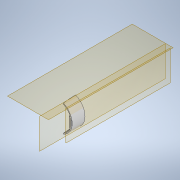
# Autodesk Inventor part: Deckel_Parachute_5_2
Saved by Autodesk Inventor 2020 (Build 240168000, 168)
## iProperties
Created: 2022-01-25
Part Number: Deckel_Parachute_5_2
Material: Generisch
Document SubType Name: Modeling
Designer: sp
Density: 1 g/cm^3
Appearance: Vorgabe
Author: sp
## iProperties of the stored document _3D-Druck.ipt
Created: 2022-05-02
Part Number: _3D-Druck
Material: Generisch
Document SubType Name: Modeling
Designer: sp
Density: 1 g/cm^3
Appearance: Vorgabe
Author: sp
Autodesk Inventor part; units mm, degrees
ref_plane "XY Plane" through (0, 0, 0) normal (0, 0, 1) x (1, 0, 0)
sketch "Skizze1" plane through (0, 0, 0) normal (0, 0, 1) x (1, 0, 0)
  circle A0 centre (0, 0) radius 31
  circle A1 centre (0, 0) radius 29
  dimension "d0" = 62
  dimension "d1" = 58
  constraints: 2 centre point, 2 coincident
  measures "d0" diameter of A0
  measures "d1" diameter of A1
extrude "Extrusion1" add sketch "Skizze1" along normal mid plane 300
sketch "Skizze2" plane through (0, 0, 0) normal (0, 1, 0) x (-1, 0, 0)
  line L0 (-11, 169.5773) -> (-11, -169.8146) construction
  line L1 (-74.8376, 0) -> (82.6362, 0) construction
  line L2 (-11, 75) -> (-11, -75)
  line L3 (-31, -150) -> (-31, 150) projected
  line L4 (31, 150) -> (-31, 150) projected
  line L5 (-31, -150) -> (31, -150) projected
  spline S0 degree 2 poles (-11, 75) (-17.8298, 136.4739) (-72.8449, 128.3193) knots 0 0 0 1 1 1
  spline S1 degree 2 poles (-11, -75) (-17.6171, -136.2673) (-74.8376, -130) knots 0 0 0 1 1 1
  line L6 (-72.8449, 128.3193) -> (-74.8376, -130)
  line L7 (-31, 120) -> (-31, 150)
  line L8 (-31, 150) -> (31, 150)
  line L9 (31, 150) -> (31, -150)
  line L10 (31, -150) -> (31, 150) projected
  line L11 (31, -150) -> (-31, -150)
  line L12 (-31, -150) -> (-31, -120)
  point P0 (0, 0)
  dimension "d4" = 11
  dimension "d5" = 150
  dimension "d6" = 30
  dimension "d7" = 30
  constraints: 18 end point, 5 point on line, 3 perpendicular, 2 collinear, 1 horizontal, 1 symmetric about line, 1 vertical, 6 other
  measures "d4" distance from line of point (0, 0) L0
  measures "d5" distance of L2.start L2.end
  measures "d6" distance from line of L7.start L4
  measures "d7" distance from line of L12.end L5
extrude "Extrusion3" cut sketch "Skizze2" along normal mid plane 100 contours S0 L3 L4 L9 L5 S1 L2
ref_plane "Arbeitsebene3" through (0, 33.25, 0) normal (0, 1, 0) x (-1, 0, 0)
sketch "Skizze8" plane through (0, 33.25, 0) normal (0, 1, 0) x (-1, 0, 0)
  line L0 (-11, -75) -> (-11, 75) projected
  arc A0 (-11, 56.4646) -> (-14.2842, 92.4804) centre (-300.1138, 48.2584) ccw
  arc A1 (-11, 56.4646) -> (-14.2842, 92.4804) centre (-31.6354, 72.7405) ccw
  point P0 (0, 0)
  constraints: 4 point on circle, 2 centre point, 1 point on line
extrude "Extrusion6" cut sketch "Skizze8" against normal blind 65
mirror "Spiegeln2" about plane through (0, 0, 0) normal (0, 0, 1) of "Extrusion6"
ref_plane "Arbeitsebene7" through (15, 0, 0) normal (1, 0, 0) x (0, 1, 0)
sketch "Skizze16" plane through (15, 0, 0) normal (1, 0, 0) x (0, 1, 0)
  line L0 (80.6197, 79.5) -> (-53.6874, 79.5) construction
  line L1 (57.2311, 79.5) -> (-60.0661, 79.5)
  line L2 (-60.0661, 79.5) -> (-60.0661, 136.8193)
  line L3 (-60.0661, 136.8193) -> (57.2311, 136.8193)
  line L4 (57.2311, 136.8193) -> (57.2311, 79.5)
  point P0 (0, 0)
  point P1 (0, 120)
  dimension "d83" = 40.5
  constraints: 10 end point, 2 horizontal, 2 parallel, 1 perpendicular, 1 point on line
  measures "d83" distance from line of point (0, 120) L0
extrude "Extrusion15" cut sketch "Skizze16" against normal mid plane 35
ref_plane "Arbeitsebene8" through (27.75, 0, 0) normal (1, 0, 0) x (0, 1, 0)
sketch "Skizze17" plane through (27.75, 0, 0) normal (1, 0, 0) x (0, 1, 0)
  line L0 (0, 106.4673) -> (0, -19.1283) construction
  line L1 (26.1314, 79.5) -> (-26.1314, 79.5) projected
  line L2 (11, 79.5) -> (-11, 79.5)
  line L3 (-11, 79.5) -> (-11, 67.5)
  line L4 (-11, 67.5) -> (11, 67.5)
  line L5 (11, 67.5) -> (11, 79.5)
  point P0 (0, 0)
  dimension "d87" = 12
  dimension "d88" = 22
  constraints: 10 end point, 2 parallel, 2 point on line, 1 horizontal, 1 perpendicular, 1 vertical, 1 other
  measures "d87" distance of L2.end L3.end
  measures "d88" distance of L3.end L4.end
extrude "Extrusion16" add sketch "Skizze17" against normal blind 3
sketch "Skizze18" plane through (15, 0, 0) normal (1, 0, 0) x (0, 1, 0)
  line L0 (36.302, 52.5896) -> (-53.6938, 52.5896)
  line L1 (-53.6938, 52.5896) -> (-53.6938, -134.0275)
  line L2 (-53.6938, -134.0275) -> (36.302, -134.0275)
  line L3 (36.302, -134.0275) -> (36.302, 52.5896)
  point P0 (0, 0)
  constraints: 8 end point, 2 parallel, 1 horizontal, 1 perpendicular
extrude "Extrusion17" cut sketch "Skizze18" along normal mid plane 35
